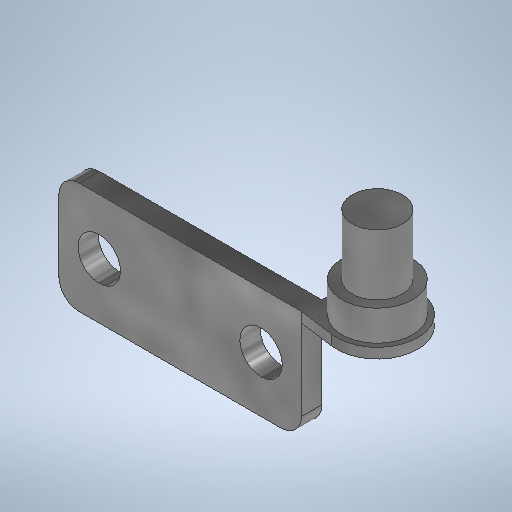
# Autodesk Inventor part: hinge
Saved by Autodesk Inventor 2025.1 (Build 291241020, 241B)
## iProperties
Created: 2024-01-14
Part Number: hinge
Material: 一般
Document SubType Name: Modeling
Designer: 8326d
Density: 1 g/cm^3
Appearance: 鋼材 メッキ
Author: 8326d
Autodesk Inventor part; units mm, degrees
ref_plane "YZ Plane" through (0, 0, 0) normal (1, 0, 0) x (0, 1, 0)
ref_plane "XZ Plane" through (0, 0, 0) normal (0, 1, 0) x (-1, 0, 0)
ref_plane "XY Plane" through (0, 0, 0) normal (0, 0, 1) x (1, 0, 0)
sketch "スケッチ1" plane through (0, 0, 0) normal (0, 0, 1) x (1, 0, 0)
  line L0 (-6, -2.75) -> (6, -2.75)
  line L1 (6, -2.75) -> (6, 2.75)
  line L2 (6, 2.75) -> (-6, 2.75)
  line L3 (-6, 2.75) -> (-6, -2.75)
  line L4 (-6, -2.75) -> (6, 2.75) construction
  line L5 (6, -2.75) -> (-6, 2.75) construction
  point P0 (0, 0)
  point P1 (0, 0)
  point P2 (0, 0)
  dimension "d0" = 12
  dimension "d1" = 5.5
  constraints: 12 end point, 3 midpoint, 2 parallel, 1 coincident, 1 horizontal, 1 perpendicular
  measures "d0" distance of L2.end L1.end
  measures "d1" distance of L1.end L0.end
extrude "押し出し1" add sketch "スケッチ1" along normal mid plane 1
sketch "スケッチ2" plane through (-6, 2.75, 0.5) normal (0, 1, 0) x (1, 0, 0)
  circle A0 centre (14, 1.75) radius 1.75
  line L0 (12, 0) -> (0, 0) projected
  line L1 (12, 1) -> (12, 0) projected
  circle A1 centre (14, 1.75) radius 2
  line L2 (12, 0) -> (13.7345, -0.2323)
  line L3 (12, 1) -> (12, 1.75)
  point P0 (6, 0.5)
  dimension "d4" = 3.5
  dimension "d5" = 4
  constraints: 4 end point, 3 tangent, 2 centre point, 2 point on circle, 1 coincident, 1 vertical
  measures "d4" diameter of A0
  measures "d5" diameter of A1
extrude "押し出し2" add sketch "スケッチ2" against normal blind 0.5 contours A0 | L3 A1 L2 L1 | A1
sketch "スケッチ3" plane through (-6, 2.75, 0.5) normal (0, 1, 0) x (1, 0, 0)
  arc A0 (13.7345, -0.2323) -> (12, 1.75) centre (14, 1.75) ccw projected
  circle A1 centre (14, 1.75) radius 1.75
  point P0 (6, 0.5)
  dimension "d8" = 3.5
  constraints: 1 centre point, 1 coincident
  measures "d8" diameter of A1
extrude "押し出し3" add sketch "スケッチ3" along normal blind 1.5
sketch "スケッチ4" plane through (8, 4.25, -1.25) normal (0, 1, 0) x (1, 0, 0)
  circle A0 centre (0, 0) radius 1.25
  circle A1 centre (0, 0) radius 1.75 projected
  point P0 (-8, -1.25)
  dimension "d11" = 2.5
  constraints: 1 centre point, 1 coincident
  measures "d11" diameter of A0
extrude "押し出し4" add sketch "スケッチ4" along normal blind 3 contours A0
sketch "スケッチ5" plane through (0, 0, 0.5) normal (0, 0, 1) x (1, 0, 0)
  line L0 (-6, 2.75) -> (-6, -2.75) projected
  line L1 (6, -2.75) -> (6, 2.25) projected
  line L2 (-6, 0) -> (6, 0) construction
  point P0 (0, 0)
  point P1 (-4, 0)
  point P2 (4, 0)
  point P3 (0, 0)
  dimension "d14" = 4
  dimension "d15" = 4
  constraints: 3 point on line, 2 end point, 2 midpoint, 1 perpendicular
  measures "d14" distance of point (0, 0) point (-4, 0)
  measures "d15" distance of point (0, 0) point (4, 0)
hole "穴1" at (-4, 0, 0.5) at (4, 0, 0.5) direction (0, 0, -1) diameter 2.1 depth 4 tip angle 118
fillet "フィレット1" radius 1 3 edges at (6, -2.75, 0) (-6, -2.75, 0) (-6, 2.75, 0)
equation "\"d15\" = d14"
